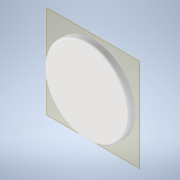
# Autodesk Inventor part: totmannschalter_deckel
Saved by Autodesk Inventor 2021.3 (Build 253353010, 353A)
## iProperties
Created: 2021-08-03
Part Number: totmannschalter_deckel
Material: Generisch
Document SubType Name: Modeling
Designer: Markus
Density: 1 g/cm^3
Appearance: Vorgabe
Author: Markus
Autodesk Inventor part; units mm, degrees
ref_plane "YZ Plane" through (0, 0, 0) normal (1, 0, 0) x (0, 1, 0)
ref_plane "XZ Plane" through (0, 0, 0) normal (0, 1, 0) x (-1, 0, 0)
ref_plane "Arbeitsebene1" through (0, 0, 0) normal (0, 0, 1) x (1, 0, 0)
sketch "Skizze1" plane through (0, 0, 0) normal (0, 0, 1) x (1, 0, 0)
  arc A0 (20.5477, -9.1676) -> (20.5477, 9.1676) centre (0, 0) ccw projected
  arc A1 (20.5477, 9.1676) -> (-20.5477, 9.1676) centre (0, 0) ccw projected
  arc A2 (-20.5477, 9.1676) -> (-20.5477, -9.1676) centre (0, 0) ccw projected
  arc A3 (-20.5477, -9.1676) -> (20.5477, -9.1676) centre (0, 0) ccw projected
  circle A4 centre (0, 0) radius 21.25 projected
  circle A5 centre (0, 0) radius 21.35
  dimension "d0" = 0.1
  constraints: 1 centre point
  measures "d0" radial gap between concentric circles of A4 A5
ref_plane "Arbeitsebene2" through (-21.25, -21.25, 1.8) normal (0, 0, 1) x (1, 0, 0)
extrude "Extrusion1" add sketch "Skizze1" along normal up to surface (1.8 mm away) contours A3 A2 A1 A0
sketch "Skizze2" plane through (0, 0, 1.8) normal (0, 0, 1) x (1, 0, 0)
  circle A0 centre (0, 0) radius 22.5
  constraints: 1 centre point, 1 coincident
extrude "Extrusion2" add sketch "Skizze2" along normal blind 1.6
fillet "Rundung1" radius 1 1 edges at (-22.5, 0, 3.4)
